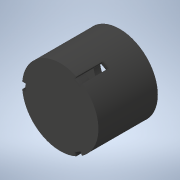
# Autodesk Inventor part: Magnetic Encoder
Saved by Autodesk Inventor 2021.4 (Build 254397000, 397)
## iProperties
Created: 2020-05-14
Part Number: Magnetic Encoder
Material: Polylactid (PLA) black
Document SubType Name: Modeling
Designer: Alex
Density: 1.3 g/cm^3
Appearance: Generic
Mass: 3.49049 g
Surface Area: 35.3155 cm^2
Volume: 2.68499 cm^3
MEncoder_FixationHole_Dia: 17,000 mm
MEncoder_OuterDia: 23,000 mm
MagneticEnc_Magnet_PassHole: 12,000 mm
Author: Alex
Autodesk Inventor part; units mm, degrees
ref_plane "YZ Plane" through (0, 0, 0) normal (1, 0, 0) x (0, 1, 0)
ref_plane "XZ Plane" through (0, 0, 0) normal (0, 1, 0) x (-1, 0, 0)
ref_plane "XY Plane" through (0, 0, 0) normal (0, 0, 1) x (1, 0, 0)
sketch "Skizze1" plane through (0, 0, 0) normal (0, 0, 1) x (1, 0, 0)
  circle A0 centre (0, 0) radius 11.5
  circle A1 centre (0, 0) radius 8.5 construction
  circle A2 centre (0, 8.5) radius 1.15
  circle A3 centre (0, -8.5) radius 1.15
  line L0 (0, 16.1) -> (0, -16.1) construction
  circle A4 centre (0, 0) radius 6
  dimension "MEncoder_OuterDia" = 23
  dimension "MEncoder_FixationHole_Dia" = 17
  dimension "d2" = 2.3
  dimension "d3" = 2.3
  dimension "MagneticEnc_Magnet_PassHole" = 12
  constraints: 5 centre point, 3 coincident, 2 point on circle, 2 point on line
  measures "MEncoder_OuterDia" diameter of A0
  measures "MEncoder_FixationHole_Dia" diameter of A1
  measures "d2" diameter of A2
  measures "d3" diameter of A3
  measures "MagneticEnc_Magnet_PassHole" diameter of A4
extrude "Montageplatte" add sketch "Skizze1" along normal blind 2
sketch "Skizze2" plane through (0, 0, 2) normal (0, 0, 1) x (1, 0, 0)
  line L0 (-10.4523, 1) -> (-11.4564, 1)
  line L1 (-11.4564, -1) -> (-10.4523, -1)
  line L2 (-10.4523, 1) -> (-11.5781, -1) construction
  line L3 (-11.5781, 1) -> (-10.4523, -1) construction
  line L4 (-16.1937, 0) -> (16.1156, 0) construction
  circle A0 centre (0, 0) radius 11.5 construction
  circle A1 centre (0, 0) radius 11.5 construction
  arc A2 (-11.4564, 1) -> (-11.4564, -1) centre (0, 0) ccw
  circle A3 centre (0, 0) radius 10.5 construction
  arc A4 (-10.4523, 1) -> (-10.4523, -1) centre (0, 0) ccw
  line L5 (4.3601, -9.5519) -> (4.8622, -10.4216)
  line L6 (6.5942, -9.4216) -> (6.0922, -8.5519)
  line L7 (4.3601, -9.5519) -> (6.6551, -9.5269) construction
  line L8 (4.923, -10.5269) -> (6.0922, -8.5519) construction
  arc A5 (4.8622, -10.4216) -> (6.5942, -9.4216) centre (0, 0) ccw
  arc A6 (4.3601, -9.5519) -> (6.0922, -8.5519) centre (0, 0) ccw
  line L9 (6.0922, 8.5519) -> (6.5942, 9.4216)
  line L10 (4.8622, 10.4216) -> (4.3601, 9.5519)
  line L11 (6.0922, 8.5519) -> (4.923, 10.5269) construction
  line L12 (6.6551, 9.5269) -> (4.3601, 9.5519) construction
  arc A7 (6.5942, 9.4216) -> (4.8622, 10.4216) centre (0, 0) ccw
  arc A8 (6.0922, 8.5519) -> (4.3601, 9.5519) centre (0, 0) ccw
  point P0 (-11.0152, 0)
  point P1 (-11.0152, 0)
  point P2 (-11.0152, 0)
  point P3 (-11.5, 0)
  point P4 (5.5076, -9.5394)
  point P5 (5.5076, -9.5394)
  point P6 (5.5076, -9.5394)
  point P7 (5.75, -9.9593)
  point P8 (5.5076, 9.5394)
  point P9 (5.5076, 9.5394)
  point P10 (5.5076, 9.5394)
  point P11 (5.75, 9.9593)
  dimension "d10" = 2
  dimension "d17" = 2
  dimension "d24" = 1
  dimension "d25" = 1
  dimension "d36" = 21
  dimension "d39" = 360
  constraints: 24 end point, 17 point on circle, 8 midpoint, 7 centre point, 2 coincident, 2 point on line, 1 concentric, 1 horizontal, 1 parallel, 55 other
  measures "d10" distance of L3.start L2.end
  measures "d17" distance of L0.start L1.end
  measures "d24" distance from line of L0 point (-11.015, 0)
  measures "d25" distance between parallel lines of L1 L4
  measures "d36" diameter of A3
extrude "Schnaphebel" add sketch "Skizze2" along normal blind 8
sketch "Skizze3" plane through (0, 0, 2) normal (0, 0, 1) x (1, 0, 0)
  circle A0 centre (0, 0) radius 10.5
  line L0 (4.8622, -10.4216) -> (4.3601, -9.5519) projected
  arc A1 (4.3601, -9.5519) -> (6.0922, -8.5519) centre (0, 0) ccw projected
  line L1 (6.0922, -8.5519) -> (6.5942, -9.4216) projected
  arc A2 (6.5942, -9.4216) -> (6.5942, 9.4216) centre (0, 0) ccw projected
  line L2 (6.5942, 9.4216) -> (6.0922, 8.5519) projected
  arc A3 (6.0922, 8.5519) -> (4.3601, 9.5519) centre (0, 0) ccw projected
  line L3 (4.3601, 9.5519) -> (4.8622, 10.4216) projected
  arc A4 (4.8622, 10.4216) -> (-11.4564, 1) centre (0, 0) ccw projected
  line L4 (-11.4564, 1) -> (-10.4523, 1) projected
  arc A5 (-10.4523, 1) -> (-10.4523, -1) centre (0, 0) ccw projected
  line L5 (-10.4523, -1) -> (-11.4564, -1) projected
  arc A6 (-11.4564, -1) -> (4.8622, -10.4216) centre (0, 0) ccw projected
  circle A7 centre (0, 8.5) radius 1.15 projected
  circle A8 centre (0, -8.5) radius 1.15 projected
  circle A9 centre (0, 0) radius 6 projected
  dimension "d41" = 21
  constraints: 1 centre point, 1 coincident
  measures "d41" diameter of A0
extrude "Sensorabdeckung" add sketch "Skizze3" along normal blind 16 contours A0 L2 A2 L1 | A0 L4 A4 L3 | L0 A6 L5 A0
sketch "Skizze4" plane through (0, 0, 18) normal (0, 0, 1) x (1, 0, 0)
  circle A0 centre (0, 0) radius 10.5
  arc A1 (4.3601, 9.5519) -> (-10.4523, 1) centre (0, 0) ccw projected
  constraints: 1 centre point, 1 concentric
extrude "Sensorabdeckung Deckel" add sketch "Skizze4" against normal blind 3
